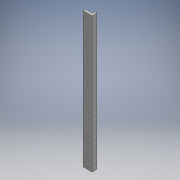
# Autodesk Inventor part: MCbeam
Saved by Autodesk Inventor 2016 (Build 200138000, 138)
## iProperties
Created: 2015-09-04
Part Number: MCbeam
Material: Generic
Document SubType Name: Modeling
Designer: Tim
Density: 1 g/cm^3
Appearance: Default
Author: Tim
Autodesk Inventor part; units mm, degrees
ref_plane "YZ Plane" through (0, 0, 0) normal (1, 0, 0) x (0, 1, 0)
ref_plane "XZ Plane" through (0, 0, 0) normal (0, 1, 0) x (-1, 0, 0)
ref_plane "XY Plane" through (0, 0, 0) normal (0, 0, 1) x (1, 0, 0)
sketch "Sketch1" plane through (0, 0, 0) normal (0, 1, 0) x (-1, 0, 0)
  line L0 (-13.5, 208) -> (13.5, 208)
  line L1 (13.5, 208) -> (13.5, -208)
  line L2 (13.5, -208) -> (-13.5, -208)
  line L3 (-13.5, -208) -> (-13.5, 208)
  line L4 (-13.5, 208) -> (13.5, -208) construction
  line L5 (13.5, 208) -> (-13.5, -208) construction
  circle A0 centre (0, 200) radius 1.85 projected
  circle A1 centre (0, 184) radius 1.85 projected
  circle A2 centre (0, 168) radius 1.85 projected
  circle A3 centre (0, 152) radius 1.85 projected
  circle A4 centre (0, 136) radius 1.85 projected
  circle A5 centre (0, 120) radius 1.85 projected
  circle A6 centre (0, 104) radius 1.85 projected
  circle A7 centre (0, 88) radius 1.85 projected
  circle A8 centre (0, 72) radius 1.85 projected
  circle A9 centre (0, 56) radius 1.85 projected
  circle A10 centre (0, 40) radius 1.85 projected
  circle A11 centre (0, 24) radius 1.85 projected
  circle A12 centre (0, 8) radius 1.85 projected
  circle A13 centre (0, 8) radius 1.85 projected
  circle A14 centre (0, -8) radius 1.85 projected
  circle A15 centre (0, -24) radius 1.85 projected
  circle A16 centre (0, -40) radius 1.85 projected
  circle A17 centre (0, -56) radius 1.85 projected
  circle A18 centre (0, -72) radius 1.85 projected
  circle A19 centre (0, -88) radius 1.85 projected
  circle A20 centre (0, -104) radius 1.85 projected
  circle A21 centre (0, -120) radius 1.85 projected
  circle A22 centre (0, -136) radius 1.85 projected
  circle A23 centre (0, -152) radius 1.85 projected
  circle A24 centre (0, -168) radius 1.85 projected
  circle A25 centre (0, -184) radius 1.85 projected
  circle A26 centre (0, -200) radius 1.85 projected
  circle A27 centre (8, -192) radius 1.85 projected
  circle A28 centre (8, -128) radius 1.85 projected
  circle A29 centre (8, 192) radius 1.85 projected
  circle A30 centre (8, 128) radius 1.85 projected
  point P0 (0, 0)
  dimension "d0" = 27
  dimension "d1" = 416
  constraints: 12 end point, 2 midpoint, 2 parallel, 1 horizontal, 1 perpendicular
  measures "d0" distance of L1.end L2.end
  measures "d1" distance of L0.end L1.end
extrude "Extrusion4" add sketch "Sketch1" along normal blind 6
sketch "Sketch2" plane through (0, 6, 0) normal (0, 1, 0) x (1, 0, 0)
  line L0 (13.5, -208) -> (13.5, 208) projected
  line L1 (0, 0) -> (13.5, 0)
  line L2 (13.5, 0) -> (10.5, 0)
  line L3 (7.5, 208) -> (13.5, 208)
  line L4 (13.5, 208) -> (13.5, -208)
  line L5 (13.5, -208) -> (7.5, -208)
  line L6 (7.5, -208) -> (7.5, 208)
  line L7 (7.5, 208) -> (13.5, -208) construction
  line L8 (13.5, 208) -> (7.5, -208) construction
  dimension "d10" = 3
  dimension "d11" = 6
  constraints: 16 end point, 3 midpoint, 2 horizontal, 2 parallel, 1 coincident, 1 perpendicular, 1 point on line
  measures "d10" distance of L1.end L2.end
  measures "d11" distance of L0.start L5.end
extrude "Extrusion5" add sketch "Sketch2" along normal blind 8
body "Solid4"
